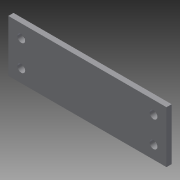
# Autodesk Inventor part: Parallel_Link_Supporter
Saved by Autodesk Inventor 2013 (Build 170138000, 138)
## iProperties
Created: 2014-03-12
Part Number: Parallel_Link_Supporter
Material: 一般
Document SubType Name: Modeling
Designer: ko
Density: 1 g/cm^3
Author: ko
Autodesk Inventor part; units mm, degrees
ref_plane "YZ Plane" through (0, 0, 0) normal (1, 0, 0) x (0, 1, 0)
ref_plane "XZ Plane" through (0, 0, 0) normal (0, 1, 0) x (-1, 0, 0)
ref_plane "XY Plane" through (0, 0, 0) normal (0, 0, 1) x (1, 0, 0)
sketch "スケッチ1" plane through (0, 0, 0) normal (0, 1, 0) x (-1, 0, 0)
  line L0 (-30.5, 10) -> (30.5, 10)
  line L1 (30.5, 10) -> (30.5, -10)
  line L2 (30.5, -10) -> (-30.5, -10)
  line L3 (-30.5, -10) -> (-30.5, 10)
  point P0 (0, 0)
  dimension "d0" = 20
  dimension "d2" = 61
  dimension "d3" = 30.5
  dimension "d4" = 10
  constraints: 8 end point, 2 parallel, 1 horizontal, 1 perpendicular
  measures "d0" distance of L2.end L0.start
  measures "d2" distance of L0.start L0.end
  measures "d3" distance from line of L1 point (0, 0)
  measures "d4" distance from line of L0 point (0, 0)
extrude "押し出し1" add sketch "スケッチ1" along normal blind 2
sketch "スケッチ2" plane through (0, 2, 0) normal (0, 1, 0) x (1, 0, 0)
  line L0 (30.5, -10) -> (30.5, 10) projected
  line L1 (30.5, 10) -> (-30.5, 10) projected
  line L2 (-30.5, 10) -> (-30.5, -10) projected
  circle A0 centre (-25.5, 5) radius 1.5
  circle A1 centre (-25.5, -5) radius 1.5
  circle A2 centre (25.5, -5) radius 1.5
  circle A3 centre (25.5, 5) radius 1.5
  point P0 (0, 0)
  dimension "d7" = 10
  dimension "d9" = 5
  dimension "d10" = 5
  dimension "d11" = 10
  dimension "d12" = 5
  dimension "d13" = 5
  dimension "d14" = 5
  dimension "d15" = 5
  dimension "d16" = 3
  constraints: 4 centre point, 3 equal radius
  measures "d7" distance of A0.centre A1.centre
  measures "d9" distance from line of L1 A0.centre
  measures "d10" distance from line of L1 A3.centre
  measures "d11" distance of A3.centre A2.centre
  measures "d12" distance from line of L2 A0.centre
  measures "d13" distance from line of L2 A1.centre
  measures "d14" distance from line of L0 A2.centre
  measures "d15" distance from line of L0 A3.centre
  measures "d16" diameter of A3
hole "穴1" at (-25.5, 2, -5) at (-25.5, 2, 5) at (25.5, 2, 5) at (25.5, 2, -5) direction (0, -1, 0) diameter 3 end through all
